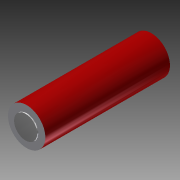
# Autodesk Inventor part: AA
Saved by Autodesk Inventor 2016 (Build 200138000, 138)
## iProperties
Created: 2015-06-28
Part Number: AA
Material: Acetal Resin, White
Document SubType Name: Modeling
Designer: Tyler
Density: 1.425 g/cm^3
Appearance: Smooth - White
Mass: 11.4589 g
Surface Area: 25.6519 cm^2
Volume: 8.0413 cm^3
Author: Tyler
Autodesk Inventor part; units mm, degrees
ref_plane "YZ Plane" through (0, 0, 0) normal (1, 0, 0) x (0, 1, 0)
ref_plane "XZ Plane" through (0, 0, 0) normal (0, 1, 0) x (-1, 0, 0)
ref_plane "XY Plane" through (0, 0, 0) normal (0, 0, 1) x (1, 0, 0)
sketch "Sketch2" plane through (0, 0, 0) normal (0, 0, 1) x (1, 0, 0)
  line L0 (0, 0) -> (-4.5, 0)
  line L1 (-4.5, 0) -> (-4.5, 0.4)
  line L2 (-4.5, 0.4) -> (-7.25, 0.4)
  line L3 (-7.25, 0.4) -> (-7.25, 48.8)
  line L4 (-7.25, 48.8) -> (-2.5, 48.8)
  line L5 (-2.5, 48.8) -> (-2.5, 50)
  line L6 (-2.5, 50) -> (0, 50)
  line L7 (0, 50) -> (0, 0)
  dimension "d0" = 50
  dimension "d1" = 7.25
  dimension "d2" = 2.5
  dimension "d3" = 1.2
  dimension "d4" = 0.4
  dimension "d5" = 4.5
  constraints: 16 end point, 4 parallel, 3 perpendicular, 1 horizontal
  measures "d0" distance between parallel lines of L0 L6
  measures "d1" distance between parallel lines of L7 L3
  measures "d2" distance of L5.end L6.end
  measures "d3" distance of L4.end L5.end
  measures "d4" distance of L0.end L1.end
  measures "d5" distance of L0.start L0.end
revolve "Revolution1" add sketch "Sketch2" angle 360 about axis through (0, 50, 0) along (0, -1, 0)
body "Solid1"
